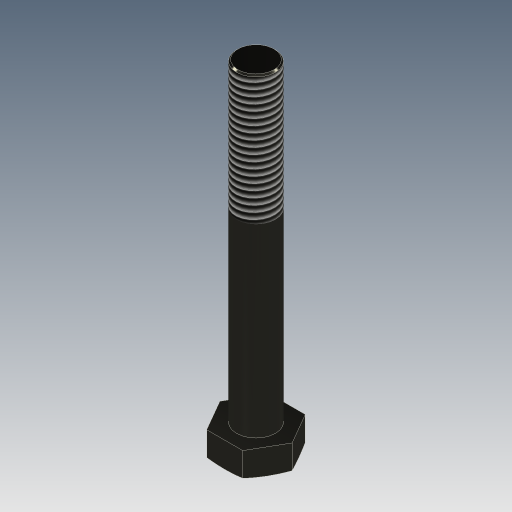
# Autodesk Inventor part: Bolt
Saved by Autodesk Inventor 2023.1 (Build 271208000, 208)
## iProperties
Created: 2023-01-24
Part Number: Bolt
Material: Acciaio
Document SubType Name: Modeling
Designer: Cominelli Nicolas
Mass: 29.04 g
Surface Area: 20.2158 cm^2
Volume: 3.69936 cm^3
Density: 7.85 g/cm^3
Appearance: Bronzo duro
Author: Cominelli Nicolas
Costo: 0
Trattamento: -
Autodesk Inventor part; units mm, degrees
ref_plane "YZ Plane" through (0, 0, 0) normal (1, 0, 0) x (0, 1, 0)
ref_plane "XZ Plane" through (0, 0, 0) normal (0, 1, 0) x (-1, 0, 0)
ref_plane "XY Plane" through (0, 0, 0) normal (0, 0, 1) x (1, 0, 0)
sketch "Schizzo4" plane through (0, 0, 0) normal (0, 0, 1) x (1, 0, 0)
  line L0 (0, 0) -> (0, 68)
  line L1 (0, 68) -> (3.9, 68)
  line L2 (3.9, 68) -> (3.9, 5.2)
  line L3 (3.9, 5.2) -> (7.5, 5.2)
  line L4 (7.5, 5.2) -> (7.5, 0)
  line L5 (7.5, 0) -> (0, 0)
  dimension "d0" = 5.2
  dimension "d1" = 7.8
  dimension "d2" = 15
  dimension "d3" = 68
  constraints: 12 end point, 4 perpendicular, 1 horizontal, 1 vertical
  measures "d0" distance of L3.end L4.end
  measures "d1" diameter of L2 L0
  measures "d2" diameter of L4 L0
  measures "d3" distance between parallel lines of L5 L1
revolve "Rivoluzione1" add sketch "Schizzo4" angle 360 about axis through (0, 0, 0) along (0, 1, 0)
thread "Filettatura1" size "M8x1.25" class "6g" standard "ANSI Metric M Profile" length 62.5 offset 37
sketch "Schizzo5" plane through (0, 0, 0) normal (0, -1, 0) x (1, 0, 0)
  line L0 (-3.6084, -6.25) -> (-7.2169, 0)
  line L1 (-7.2169, 0) -> (-3.6084, 6.25)
  line L2 (-3.6084, 6.25) -> (3.6084, 6.25)
  line L3 (3.6084, 6.25) -> (7.2169, 0)
  line L4 (7.2169, 0) -> (3.6084, -6.25)
  line L5 (3.6084, -6.25) -> (-3.6084, -6.25)
  circle A0 centre (0, 0) radius 7.5 projected
  dimension "d9" = 12.5
  constraints: 12 end point, 1 coincident, 1 horizontal, 13 other
  measures "d9" distance between parallel lines of L2 L5
extrude "Estrusione1" cut sketch "Schizzo5" against normal up to surface (5.2 mm away)
sketch "Schizzo6" plane through (0, 0, 0) normal (0, 0, 1) x (1, 0, 0)
  line L0 (3.9, 68) -> (-3.9, 68) projected
  line L1 (3.6, 68) -> (3.9, 67.7)
  line L2 (3.9, 5.2) -> (3.9, 68) projected
  line L3 (3.9, 68) -> (3.6, 68)
  line L4 (3.6084, 0) -> (7.2169, 0) projected
  line L5 (5.75, 0) -> (7.2169, 0.4)
  line L6 (7.2169, 0.4) -> (7.2169, 0)
  line L7 (7.2169, 0) -> (5.75, 0)
  line L8 (7.2169, 5.2) -> (3.6084, 5.2) projected
  line L9 (0, 0) -> (0, 68)
  dimension "d12" = 45
  dimension "d14" = 0.3
  dimension "d15" = 4.8
  dimension "d16" = 11.5
  constraints: 12 end point, 3 point on line, 2 perpendicular, 1 horizontal, 1 midpoint
  measures "d12" angle of L0 L1
  measures "d14" distance from line of L1.end L0
  measures "d15" distance from line of L5.end L8
  measures "d16" diameter of L5.start L9
revolve "Rivoluzione3" cut sketch "Schizzo6" angle 360 about axis through (0, 0, 0) along (0, 1, 0)
